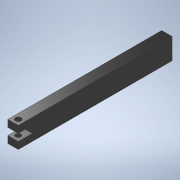
# Autodesk Inventor part: ShortBraillePlunger
Saved by Autodesk Inventor 2020.1 (Build 241239000, 239)
## iProperties
Created: 2020-02-22
Part Number: ShortBraillePlunger
Material: Generic
Document SubType Name: Modeling
Designer: Dominic
Density: 1 g/cm^3
Appearance: Glossy - Black
Author: Dominic
Autodesk Inventor part; units mm, degrees
ref_plane "YZ Plane" through (0, 0, 0) normal (1, 0, 0) x (0, 1, 0)
ref_plane "XZ Plane" through (0, 0, 0) normal (0, 1, 0) x (-1, 0, 0)
ref_plane "XY Plane" through (0, 0, 0) normal (0, 0, 1) x (1, 0, 0)
sketch "Sketch1" plane through (0, 0, 0) normal (1, 0, 0) x (0, 1, 0)
  line L0 (-9.525, -69.85) -> (9.525, -69.85)
  line L1 (9.525, -69.85) -> (9.525, 69.85)
  line L2 (9.525, 69.85) -> (-9.525, 69.85)
  line L3 (-9.525, 69.85) -> (-9.525, -69.85)
  line L4 (-9.525, -69.85) -> (9.525, 69.85) construction
  line L5 (9.525, -69.85) -> (-9.525, 69.85) construction
  point P0 (0, 0)
  dimension "d0" = 19.05
  dimension "d1" = 139.7
  constraints: 12 end point, 2 midpoint, 2 parallel, 1 horizontal, 1 perpendicular
  measures "d0" distance of L2.end L1.end
  measures "d1" distance of L0.end L1.end
extrude "Extrusion1" add sketch "Sketch1" along normal mid plane 9.525
sketch "Sketch2" plane through (4.7625, 0, 0) normal (1, 0, 0) x (0, 0, -1)
  line L0 (-82.55, -3.175) -> (-57.15, -3.175)
  line L1 (-57.15, -3.175) -> (-57.15, 3.175)
  line L2 (-57.15, 3.175) -> (-82.55, 3.175)
  line L3 (-82.55, 3.175) -> (-82.55, -3.175)
  line L4 (-69.85, 9.525) -> (-69.85, -9.525) projected
  line L5 (-82.55, -3.175) -> (-57.15, 3.175) construction
  line L6 (-57.15, -3.175) -> (-82.55, 3.175) construction
  point P0 (0, 0)
  point P1 (-69.85, 0)
  point P2 (-69.85, 3.175)
  point P3 (-69.85, -3.175)
  dimension "d4" = 6.35
  dimension "d5" = 12.7
  constraints: 12 end point, 3 midpoint, 2 parallel, 1 horizontal, 1 perpendicular
  measures "d4" distance of L0.end L1.end
  measures "d5" distance between parallel lines of L1 L4
extrude "Extrusion2" cut sketch "Sketch2" against normal blind 25.4 contours L4 L2 L1 L0
sketch "Sketch3" plane through (-4.7625, 9.525, 69.85) normal (0, 1, 0) x (1, 0, 0)
  line L0 (9.525, 0) -> (0, 0) projected
  circle A0 centre (4.7625, 4.7625) radius 2.6035
  point P0 (4.7625, 69.85)
  point P1 (4.7625, 0)
  dimension "d8" = 5.207
  dimension "d9" = 4.7625
  constraints: 1 centre point, 1 midpoint, 1 vertical alignment
  measures "d8" diameter of A0
  measures "d9" distance from line of L0 A0.centre
extrude "Extrusion3" cut sketch "Sketch3" against normal blind 6.35
sketch "Sketch4" plane through (-4.7625, 9.525, 69.85) normal (0, 1, 0) x (1, 0, 0)
  circle A0 centre (4.7625, 4.7625) radius 2.6035 projected
  circle A1 centre (4.7625, 4.7625) radius 2.3813
  point P0 (4.7625, 69.85)
  dimension "d12" = 4.7625
  constraints: 1 centre point, 1 coincident
  measures "d12" diameter of A1
extrude "Extrusion4" cut sketch "Sketch4" against normal blind 25.4 contours A1
body "Solid1"
